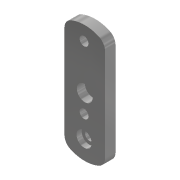
# Autodesk Inventor part: Front-Idlers_Housing-Cover
Saved by Autodesk Inventor 2021 (Build 250183000, 183)
## iProperties
Created: 2021-09-01
Part Number: Front-Idlers_Housing-Cover
Material: Generisch
Document SubType Name: Modeling
Designer: Rama
Density: 1 g/cm^3
Appearance: Glatt - Mittelgrau
Author: Rama
Autodesk Inventor part; units mm, degrees
ref_plane "YZ Plane" through (0, 0, 0) normal (1, 0, 0) x (0, 1, 0)
ref_plane "XZ Plane" through (0, 0, 0) normal (0, 1, 0) x (-1, 0, 0)
ref_plane "XY Plane" through (0, 0, 0) normal (0, 0, 1) x (1, 0, 0)
sketch "Skizze1" plane through (0, 0, 0) normal (0, 0, 1) x (1, 0, 0)
  circle A0 centre (7.5, 13) radius 1.7 projected
  circle A1 centre (7.5, 37) radius 1.7 projected
  arc A2 (15.5, 37.6806) -> (13.0863, 41.3526) centre (11.5, 37.6806) ccw projected
  arc A3 (13.0863, 41.3526) -> (2.4137, 41.3526) centre (7.75, 29) ccw projected
  arc A4 (2.4137, 41.3526) -> (0, 37.6806) centre (4, 37.6806) ccw projected
  line L0 (0, 2.3194) -> (0, 37.6806) projected
  arc A5 (0, 2.3194) -> (2.4137, -1.3526) centre (4, 2.3194) ccw projected
  arc A6 (2.4137, -1.3526) -> (13.0863, -1.3526) centre (7.75, 11) ccw projected
  arc A7 (13.0863, -1.3526) -> (15.5, 2.3194) centre (11.5, 2.3194) ccw projected
  line L1 (15.5, 2.3194) -> (15.5, 37.6806) projected
  point P0 (0, 0)
extrude "Extrusion1" add sketch "Skizze1" along normal blind 5
sketch "Skizze2" plane through (0, 0, 5) normal (0, 0, 1) x (1, 0, 0)
  arc A0 (2.4137, -1.3526) -> (13.0863, -1.3526) centre (7.75, 11) ccw projected
  arc A1 (13.0863, -1.3526) -> (15.5, 2.3194) centre (11.5, 2.3194) ccw projected
  line L0 (15.5, 2.3194) -> (15.5, 37.6806) projected
  arc A2 (15.5, 37.6806) -> (13.0863, 41.3526) centre (11.5, 37.6806) ccw projected
  arc A3 (13.0863, 41.3526) -> (2.4137, 41.3526) centre (7.75, 29) ccw projected
  arc A4 (2.4137, 41.3526) -> (0, 37.6806) centre (4, 37.6806) ccw projected
  line L1 (0, 37.6806) -> (0, 2.3194) projected
  arc A5 (0, 2.3194) -> (2.4137, -1.3526) centre (4, 2.3194) ccw projected
  circle A6 centre (7.5, 37) radius 1.7 projected
  circle A7 centre (7.5, 13) radius 1.7 projected
  line L2 (7.75, 20) -> (7.75, 20)
  line L3 (7.75, 20) -> (7.75, -2.4559)
  line L4 (7.75, -2.4559) -> (7.75, -2.4559)
  line L5 (7.75, -2.4559) -> (7.75, 20)
  point P0 (0, 0)
  point P1 (7.75, -2.4559)
  dimension "d2" = 44.9119
  dimension "d3" = 15.5
  dimension "d4" = 22.456
  dimension "d5" = 0
  constraints: 8 end point, 2 equal length, 1 horizontal, 1 midpoint, 1 perpendicular, 1 point on circle
  measures "d3" distance between parallel lines of L1 L0
  measures "d5" distance between parallel lines of L3 L5
hole "Bohrung1" at (7.75, 20, 5) direction (0, 0, -1) diameter 6.05 depth 3.1
sketch "Skizze4" plane through (0, 0, 5) normal (0, 0, 1) x (1, 0, 0)
  circle A0 centre (7.5, 4.722) radius 1.9913 projected
  point P0 (0, 0)
hole "Bohrung2" at (7.5, 4.722, 5) direction (0, 0, -1) diameter 3.3 end through all counterbore diameter 5.8 counterbore depth 2 clearance for "Inbusschraube DIN EN ISO 4762" size "M3" standard "DIN"
move faces "Verschieben1" translate (0, 0, 1) faces at (13.3835, 17.8023, 0)
sketch "Skizze6" plane through (7.75, 11, 1) normal (0, 0, -1) x (-1, 0, 0)
  circle A0 centre (-5.37, 26.9384) radius 1
  circle A1 centre (5.81, 25.1971) radius 1
  circle A2 centre (5.81, 25.1971) radius 1.2
  circle A3 centre (-5.37, 26.9384) radius 1.2
  circle A4 centre (5.87, 26.9384) radius 1
  circle A5 centre (-5.37, 26.9384) radius 1
  circle A6 centre (5.87, 26.9384) radius 1.2
  arc A7 (4.9199, 26.9621) -> (4.4911, 27.5261) centre (5.45, 27.81) ccw
  circle A8 centre (-5.37, 26.9384) radius 1
  circle A9 centre (5.37, -8.778) radius 1
  circle A10 centre (-5.37, -8.778) radius 1
  circle A11 centre (5.45, 27.81) radius 1.2
  circle A12 centre (-5.37, -8.778) radius 1.2
  circle A13 centre (5.37, -8.778) radius 1.2
  point P0 (7.75, -11)
  dimension "d37" = 2.4
  dimension "d38" = 2.4
  dimension "d44" = 2.4
  dimension "d45" = 2.4
  dimension "d46" = 2.4
  dimension "d47" = 2.4
  constraints: 14 centre point, 6 coincident, 2 point on circle, 18 other
  measures "d37" diameter of A2
  measures "d38" diameter of A3
  measures "d44" diameter of A6
  measures "d45" diameter of A11
  measures "d46" diameter of A12
  measures "d47" diameter of A13
extrude "Extrusion4" cut sketch "Skizze6" against normal blind 3 contours A0 | A11 A6 | A6 A7 A4 A11 | A11 A4 A7 A6 | A4 A11 | A3 | A9 | A10 | A12 | A13
chamfer "Fase1" distance 0.6 angle 45 4 edges at (14.32, 37.9384, 4) (3.5, 38.81, 4) (3.58, 2.222, 4) (14.32, 2.222, 4)
equation "\"d4\" = 0.5 * d2"
equation "\"d37\" = d38"
equation "\"d44\" = d38"
equation "\"d45\" = d38"
equation "\"d46\" = d38"
equation "\"d47\" = d38"
